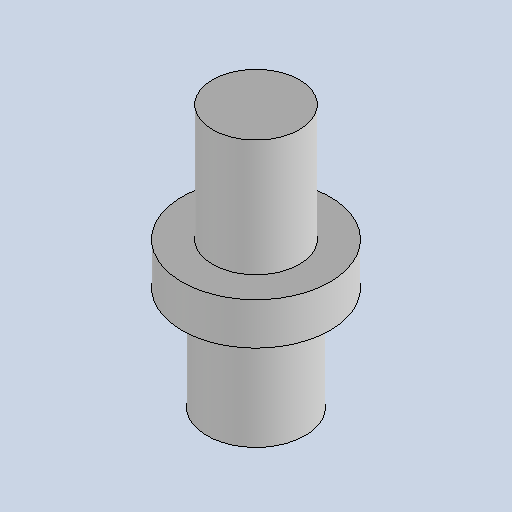
# Autodesk Inventor part: NVPH-312 augur shaft
Saved by Autodesk Inventor 2025 (Build 290162010, 162A)
## iProperties
Created: 2024-12-05
Part Number: NVPH-312 augur shaft
Material: Generic
Document SubType Name: Modeling
Designer: user
Density: 1 g/cm^3
Appearance: Default
Author: user
Autodesk Inventor part; units mm, degrees
ref_plane "XZ Plane" through (0, 0, 0) normal (0, 1, 0) x (-1, 0, 0)
ref_plane "XY Plane" through (0, 0, 0) normal (0, 0, 1) x (1, 0, 0)
sketch "Sketch2" plane through (0, 0, 0) normal (0, 1, 0) x (-1, 0, 0)
  line L0 (0, 0) -> (0, 80)
  line L1 (0, 80) -> (-13.2447, 80)
  line L2 (-13.2447, 80) -> (-13.2447, 44.3901)
  line L3 (-22.5598, 44.3901) -> (-22.5598, 31.5867)
  line L4 (-22.5598, 31.5867) -> (-15, 31.5867)
  line L5 (-15, 31.5867) -> (-15, 0)
  line L6 (-15, 0) -> (0, 0)
  line L7 (-22.5598, 44.3901) -> (-13.2447, 44.3901)
  dimension "d6" = 30
  dimension "d7" = 80
  constraints: 16 end point, 5 perpendicular, 1 horizontal, 1 parallel, 1 vertical
  measures "d6" diameter of L5 L0
  measures "d7" distance between parallel lines of L6 L1
revolve "Revolution1" add sketch "Sketch2" angle 360 about axis through (0, 0, 0) along (0, 0, 1)
ref_plane "Work Plane1" through (-13.2447, 0, 62.195) normal (1, 0, 0) x (0, 1, 0)
sketch "Sketch3" plane through (-13.2447, 0, 62.195) normal (1, 0, 0) x (0, 1, 0)
  line L0 (13.2447, -17.805) -> (-13.2447, -17.805) projected
  line L1 (13.2447, 17.805) -> (-13.2447, 17.805) projected
  line L2 (0.1403, 5.805) -> (0.1403, -4.195) construction
  line L3 (-3.8597, 5.805) -> (-3.8597, -4.195)
  line L4 (4.1403, -4.195) -> (4.1403, 5.805)
  arc A0 (4.1403, 5.805) -> (-3.8597, 5.805) centre (0.1403, 5.805) ccw
  arc A1 (-3.8597, -4.195) -> (4.1403, -4.195) centre (0.1403, -4.195) ccw
  point P0 (0, -62.195)
  point P1 (0.1403, 0.805)
  dimension "d8" = 12
  dimension "d9" = 8
  dimension "d10" = 10
  constraints: 8 end point, 4 point on circle, 4 tangent, 2 centre point, 1 midpoint, 1 parallel, 1 perpendicular, 1 vertical
  measures "d8" distance from line of L2.start L1
  measures "d9" distance between parallel lines of L4 L3
  measures "d10" distance of L2.start L2.end
extrude "Extrusion2" cut sketch "Sketch3" along normal blind 10
body "Solid2"
